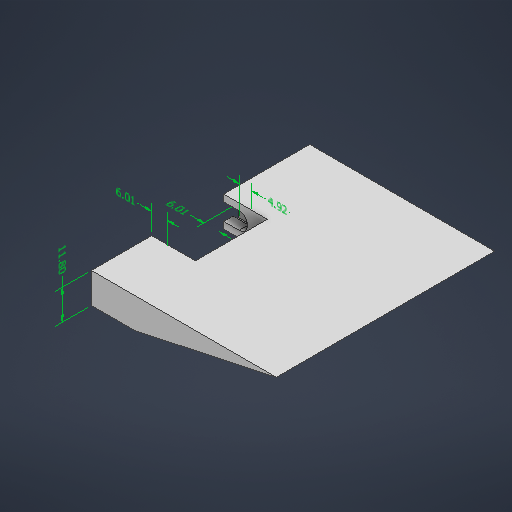
# Autodesk Inventor part: hand_right_1
Saved by Autodesk Inventor 2026.1 (Build 301233020, 233B)
## iProperties
Created: 2025-10-30
Part Number: hand_right_1
Material: Generic
Document SubType Name: Modeling
Designer: Asus
Density: 1 g/cm^3
Appearance: Default
Author: Asus
Autodesk Inventor part; units mm, degrees
ref_plane "YZ Plane" through (0, 0, 0) normal (1, 0, 0) x (0, 1, 0)
ref_plane "XZ Plane" through (0, 0, 0) normal (0, 1, 0) x (-1, 0, 0)
ref_plane "XY Plane" through (0, 0, 0) normal (0, 0, 1) x (1, 0, 0)
sketch "Sketch1" plane through (0, 0, 0) normal (0, 1, 0) x (-1, 0, 0)
  line L0 (0, 0) -> (60, 0)
  line L1 (55.02, -23.5) -> (55.02, -51.5)
  line L2 (60, -75) -> (0, -75)
  line L3 (0, -75) -> (0, 0)
  line L4 (55.02, -23.5) -> (72.02, -23.5) construction
  line L5 (72.02, -23.5) -> (72.02, -51.5) construction
  line L6 (72.02, -51.5) -> (55.02, -51.5) construction
  line L7 (55.02, -51.5) -> (55.02, -23.5)
  line L8 (72.02, -51.5) -> (55.02, -51.5)
  line L9 (60, -75) -> (72.02, -75)
  line L10 (72.02, -75) -> (72.02, -51.5)
  line L11 (72.02, -23.5) -> (55.02, -23.5)
  line L12 (60, 0) -> (72.02, 0)
  line L13 (72.02, 0) -> (72.02, -23.5)
  point P0 (55.02, -37.5)
  point P1 (63.52, -51.5)
  point P2 (63.52, -51.5)
  dimension "d2" = 28
  dimension "d25" = 8.5
  dimension "d26" = 60
  dimension "d27" = 12.02
  dimension "d28" = 72.02
  constraints: 28 end point, 6 parallel, 4 horizontal, 4 midpoint, 2 perpendicular
  measures "d2" distance of L4.end L5.end
  measures "d25" distance of L1.end point (63.52, -51.5)
  measures "d26" distance of L2.start L2.end
  measures "d27" distance of L2.start L9.end
  measures "d28" distance between parallel lines of L3 L10
extrude "Extrusion1" add sketch "Sketch1" along normal blind 11.8
sketch "Sketch2" plane through (-55.02, 0, -23.5) normal (0, 0, -1) x (-1, 0, 0)
  circle A0 centre (10.99, 5.9) radius 2
  line L0 (17, 0) -> (17, 11.8) projected
  point P0 (-55.02, 0)
  dimension "d6" = 4
  dimension "d7" = 6.01
  constraints: 1 centre point
  measures "d6" diameter of A0
  measures "d7" distance from line of L0 A0.centre
extrude "Extrusion2" cut sketch "Sketch2" against normal blind 2
sketch "Sketch3" plane through (-72.02, 0, -51.5) normal (0, 0, 1) x (1, 0, 0)
  arc A0 (6.01, 2.5893) -> (6.01, 9.1893) centre (6.01, 5.8893) ccw
  line L0 (6.01, 9.1893) -> (0, 9.1893)
  line L1 (0, 0) -> (0, 11.8) projected
  line L2 (6.01, 2.5893) -> (0, 2.5893)
  point P0 (72.02, 0)
  dimension "d10" = 6.6
  dimension "d21" = 6.01
  dimension "d22" = 6.01
  constraints: 4 end point, 2 point on circle, 2 point on line, 1 centre point, 1 horizontal, 1 parallel, 1 tangent
  measures "d10" diameter of A0
  measures "d21" distance from line of L1 A0.centre
  measures "d22" distance of L0.start L0.end
extrude "Extrusion3" cut sketch "Sketch3" against normal blind 3.65
sketch "Sketch4" plane through (-72.02, 0, -75) normal (-1, 0, 0) x (0, 0, 1)
  line L0 (19.85, 10.7643) -> (17.75, 10.7643)
  line L1 (17.75, 10.7643) -> (17.75, 1.0143)
  line L2 (17.75, 1.0143) -> (19.85, 1.0143)
  line L3 (19.85, 1.0143) -> (19.85, 10.7643)
  line L4 (19.85, 2.5893) -> (19.85, 9.1893) projected
  point P0 (75, 0)
  point P1 (19.85, 5.8893)
  dimension "d13" = 2.1
  dimension "d14" = 9.75
  constraints: 8 end point, 2 midpoint, 2 parallel, 1 horizontal, 1 perpendicular
  measures "d13" distance of L2.end L1.end
  measures "d14" distance of L0.end L1.end
extrude "Extrusion4" cut sketch "Sketch4" against normal blind 10.925
sketch "Sketch5" plane through (-72.02, 0, 0) normal (0, 0, 1) x (1, 0, 0)
  line L0 (17, 0) -> (17, 11.8) projected
  line L1 (72.02, 11.8) -> (0, 11.8) projected
  line L2 (17, 0) -> (72.02, 11.8)
  line L3 (72.02, 11.8) -> (72.02, 0)
  line L4 (72.02, 0) -> (17, 0)
  constraints: 6 end point, 2 perpendicular
extrude "Extrusion5" cut sketch "Sketch5" against normal blind 88.5 contours L2 L3 L4
sketch "Sketch6" plane through (-72.02, 0, -75) normal (0, 0, -1) x (-1, 0, 0)
  line L0 (-72.02, 11.8) -> (-17, 0) projected
  line L1 (0, 11.8) -> (-72.02, 11.8) projected
  line L2 (-72.02, 11.8) -> (0, 11.8)
  line L3 (0, 11.8) -> (0, 0)
  line L4 (-17, 0) -> (-17, 11.8) projected
  line L5 (0, 0) -> (-17, 0)
  line L6 (-17, 0) -> (-72.02, 11.8)
  point P0 (-72.02, 0)
  constraints: 8 end point, 2 perpendicular, 1 collinear
extrude "Extrusion6" add sketch "Sketch6" along normal blind 10
body "Solid1"
